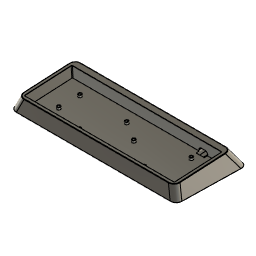
Menhirvan (Autodesk Fusion 360 design; units mm, degrees)
Autodesk Fusion 360 part; units mm, degrees
sketch "Top Plane Sketch" plane through (0, 0, 0) normal (0, 0, 1) x (1, 0, 0)
  line L0 (-95.25, -40.4812) -> (147.6375, -40.4812) construction
  line L1 (147.6375, -40.4812) -> (147.6375, 35.7188) construction
  line L2 (147.6375, 35.7188) -> (-95.25, 35.7188) construction
  line L3 (-95.25, 35.7188) -> (-95.25, -40.4813) construction
  line L4 (-95.75, -40.9812) -> (148.1375, -40.9812)
  line L5 (148.1375, -40.9812) -> (148.1375, 36.2188)
  line L6 (148.1375, 36.2188) -> (-95.75, 36.2188)
  line L7 (-95.75, 36.2188) -> (-95.75, -40.9812)
  line L8 (-100.75, -45.9812) -> (153.1375, -45.9812)
  line L9 (153.1375, -45.9812) -> (153.1375, 46.2188)
  line L10 (153.1375, 46.2188) -> (-100.75, 46.2188)
  line L11 (-100.75, 46.2188) -> (-100.75, -45.9812)
  line L12 (-95.25, 35.7188) -> (147.6375, -40.4813) construction
  line L13 (147.6375, 35.7188) -> (-95.25, -40.4813) construction
  circle A0 centre (26.1938, -2.3813) radius 1.8249 construction
  dimension "d1" = 242.8875
  dimension "d2" = 76.2
  dimension "d3" = 0.5
  dimension "d9" = 10
  dimension "d10" = 5
  dimension "d11" = 5
  dimension "d12" = 5
  constraint horizontal L0
  constraint vertical L1
  constraint horizontal L2
  constraint vertical L3
  constraint midpoint L12 A0.centre
  measures "d1" distance of L0.start L0.end
  measures "d2" distance of L0.start L2.end
  measures "d9" distance of L6 L10
  measures "d10" distance of L7 L11
  measures "d11" distance of L5 L9
  measures "d12" distance of L4 L8
ref_plane "WorkPlane1" through (0, 0, -50) normal (0, 0, 1) x (1, 0, 0)
sketch "Base Plane Sketch" plane through (0, 0, -50) normal (0, 0, 1) x (1, 0, 0)
  line L0 (147.6375, -35.7188) -> (-95.25, -35.7188) construction
  line L1 (-95.25, -35.7188) -> (-95.25, 40.4813) construction
  line L2 (-95.25, 40.4812) -> (147.6375, 40.4812) construction
  line L3 (147.6375, 40.4812) -> (147.6375, -35.7187) construction
  line L4 (147.6375, -35.7188) -> (-95.25, 40.4812) construction
  line L5 (-95.25, -35.7188) -> (147.6375, 40.4813) construction
  circle A0 centre (26.1938, 2.3812) radius 6.9017 construction
  line L6 (148.1375, -36.2188) -> (-95.75, -36.2188) construction
  line L7 (-95.75, -36.2188) -> (-95.75, 40.9812) construction
  line L8 (-95.75, 40.9812) -> (148.1375, 40.9812) construction
  line L9 (148.1375, 40.9812) -> (148.1375, -36.2188) construction
  line L10 (-100.75, 50.9812) -> (153.1375, 50.9812) construction
  line L11 (153.1375, 50.9812) -> (153.1375, -41.2188) construction
  line L12 (153.1375, -41.2188) -> (-100.75, -41.2188) construction
  line L13 (-100.75, -41.2188) -> (-100.75, 50.9812) construction
  line L14 (-120.75, 74.9813) -> (173.1375, 74.9813)
  line L15 (173.1375, 74.9813) -> (173.1375, -61.2188)
  line L16 (173.1375, -61.2188) -> (-120.75, -61.2188)
  line L17 (-120.75, -61.2188) -> (-120.75, 74.9813)
  point P0 (26.1938, 2.3812)
  dimension "d14" = 242.8875
  dimension "d15" = 76.2
  dimension "d16" = -0.5
  dimension "d17" = 10
  dimension "d18" = 5
  dimension "d19" = 5
  dimension "d20" = 5
  dimension "d21" = 20
  dimension "d22" = 20
  dimension "d23" = 20
  dimension "d24" = 24
  constraint horizontal L0
  constraint perpendicular L0 L1
  constraint parallel L0 L2
  constraint parallel L1 L3
  constraint coincident L4 P0
  constraint coincident L5 P0
  constraint coincident P0 A0.centre
  constraint horizontal L10
  constraint vertical L11
  constraint horizontal L12
  constraint vertical L13
  constraint horizontal L14
  constraint vertical L15
  constraint horizontal L16
  constraint vertical L17
  measures "d14" distance of L2.start L2.end
  measures "d15" distance of L0.end L2.start
  measures "d17" distance of L8 L10
  measures "d18" distance of L7 L13
  measures "d19" distance of L9 L11
  measures "d20" distance of L6 L12
  measures "d21" distance of L12 L16
  measures "d22" distance of L11 L15
  measures "d23" distance of L13 L17
  measures "d24" distance of L10 L14
loft "Loft1" add profiles "Top Plane Sketch", "Base Plane Sketch" section 1 section 2
sketch "Angle Cut Line" plane through (0, -42.0738, 12.822) normal (0, -0.956567, 0.291514) x (1, 0, 0)
  line L0 (153.1375, -13.4042) -> (-100.75, -13.4042)
  line L1 (-100.75, -13.4042) -> (-120.75, -65.6744)
  line L2 (-120.75, -65.6744) -> (173.1375, -65.6744)
  line L3 (173.1375, -65.6744) -> (153.1375, -13.4042)
  line L4 (-108.7852, -34.4042) -> (161.1727, -34.4042)
  dimension "d37" = 21
  constraint coincident L1 L4.start
  constraint coincident L3 L4.end
  constraint parallel L2 L4
  measures "d37" distance of L0 L4
ref_plane "WorkPlane2" through (26.1938, -52.103, -20.0879) normal (0, 0.052336, 0.99863) x (1, 0, 0)
extrude "Extrude1" cut 1 faces at (75.175, -15.8188, -50) along direction (0, 0, -1) up to surface end surface through (26.1938, -52.103, -20.0879) normal (0, 0.052336, 0.99863) offset 0
fillet "Fillet1" radius 10 4 edges at (-105.9551, 53.7043, -13.0127) (-104.7676, -49.0421, -10.0439) (157.1551, -49.0421, -10.0439) (158.3426, 53.7043, -13.0127)
extrude "Extrude2" cut sketch "Top Plane Sketch" against normal blind 18.06 contours L4 L5 L6 L7
sketch "USB C Hole" plane through (0, 36.2188, 0) normal (0, -1, 0) x (1, 0, 0)
  line L0 (-95.75, -18.06) -> (148.1375, -18.06)
  line L1 (124.347, -12.15) -> (110.397, -12.15)
  line L2 (110.397, -12.15) -> (110.397, -20.31)
  line L3 (110.397, -20.31) -> (124.347, -20.31)
  line L4 (124.347, -20.31) -> (124.347, -12.15)
  line L5 (124.347, -12.15) -> (110.397, -20.31) construction
  line L6 (110.397, -12.15) -> (124.347, -20.31) construction
  line L7 (148.1375, 0) -> (-95.75, 0)
  line L8 (-95.75, 0) -> (-95.75, -18.06)
  line L9 (148.1375, -18.06) -> (148.1375, 0)
  line L10 (-95.75, -18.06) -> (-86.225, -18.06) construction
  line L11 (-86.225, -18.06) -> (117.372, -18.06) construction
  line L12 (117.372, -18.06) -> (117.372, -16.23) construction
  point P0 (117.372, -16.23)
  dimension "d61" = 13.95
  dimension "d62" = 8.16
  dimension "d80" = 9.525
  dimension "d81" = 203.597
  dimension "d82" = 1.83
  constraint horizontal L1
  constraint perpendicular L1 L2
  constraint parallel L1 L3
  constraint parallel L2 L4
  constraint coincident L5 P0
  constraint coincident L6 P0
  constraint coincident L0.start L8.end
  constraint perpendicular L8 L10
  constraint parallel L0 L11
  constraint perpendicular L0 L12
  measures "d61" distance of L2.end L3.end
  measures "d62" distance of L1.end L2.end
  measures "d80" distance of L0.start L10.end
  measures "d81" distance of L10.end L11.end
  measures "d82" distance of L11.end P0
sketch "Screw Post Sketch" plane through (0, 0, -18.06) normal (0, 0, 1) x (1, 0, 0)
  circle A0 centre (-64.425, 17.1688) radius 2.75
  circle A1 centre (114.825, 19.2948) radius 2.75
  circle A2 centre (86.575, -29.3402) radius 2.75
  circle A3 centre (-66.025, -15.6052) radius 2.75
  circle A4 centre (-64.425, 17.1688) radius 1.6
  circle A5 centre (-66.025, -15.6052) radius 1.6
  circle A6 centre (114.825, 19.2948) radius 1.6
  circle A7 centre (86.575, -29.3402) radius 1.6
  line L0 (-95.75, -40.9812) -> (148.1375, -40.9812)
  line L1 (148.1375, -40.9812) -> (148.1375, 36.2188)
  line L2 (148.1375, 36.2188) -> (-95.75, 36.2188)
  line L3 (-95.75, 36.2188) -> (-95.75, -40.9812)
  line L4 (-95.75, 36.2188) -> (-86.225, 36.2188) construction
  line L5 (-86.225, 36.2188) -> (-86.225, 26.6938) construction
  line L6 (-86.225, 26.6938) -> (-95.75, 26.6938) construction
  line L7 (-95.75, 26.6938) -> (-95.75, 36.2188) construction
  circle A8 centre (-19.075, -29.0552) radius 2.75
  circle A9 centre (-19.075, -29.0552) radius 1.6
  circle A10 centre (42.425, -1.8812) radius 2.75
  circle A11 centre (42.425, -1.8812) radius 1.6
  circle A12 centre (11.775, 17.1688) radius 2.75
  circle A13 centre (11.775, 17.1688) radius 1.6
  dimension "d41" = 5.5
  dimension "d52" = 3.2
  dimension "d53" = 3.2
  dimension "d54" = 3.2
  dimension "d55" = 3.2
  dimension "d83" = 9.525
  dimension "d84" = 9.525
  dimension "d91" = 21.8
  dimension "d92" = 9.525
  dimension "d93" = 20.2
  dimension "d94" = 42.299
  dimension "d97" = 5.5
  dimension "d98" = 55.749
  dimension "d99" = 67.15
  dimension "d100" = 3.2
  dimension "d101" = 7.399
  dimension "d102" = 201.05
  dimension "d103" = 56.034
  dimension "d104" = 5.5
  dimension "d105" = 128.65
  dimension "d106" = 28.575
  dimension "d107" = 3.2
  dimension "d108" = 5.5
  dimension "d109" = 9.525
  dimension "d110" = 98
  dimension "d111" = 3.2
  dimension "d112" = 172.8
  constraint equal A0 A1
  constraint equal A0 A3
  constraint equal A0 A2
  constraint concentric A0 A4
  constraint concentric A3 A5
  constraint concentric A1 A6
  constraint concentric A2 A7
  constraint horizontal L4
  constraint vertical L5
  constraint horizontal L6
  constraint vertical L7
  constraint coincident L2.end L3.start
  constraint concentric A8 A9
  constraint concentric A10 A11
  constraint concentric A12 A13
  measures "d41" diameter of A0
  measures "d52" diameter of A4
  measures "d53" diameter of A5
  measures "d54" diameter of A6
  measures "d55" diameter of A7
  measures "d83" distance of L2.end L4.end
  measures "d84" distance of L2.end L6.end
  measures "d91" distance of A0.centre L5
  measures "d92" distance of A0.centre L6
  measures "d93" distance of A3.centre L5
  measures "d94" distance of A3.centre L6
  measures "d97" diameter of A8
  measures "d98" distance of L6 A8.centre
  measures "d99" distance of L5 A8.centre
  measures "d100" diameter of A9
  measures "d101" distance of A1.centre L6
  measures "d102" distance of A1.centre L5
  measures "d103" distance of A2.centre L6
  measures "d104" diameter of A10
  measures "d105" distance of L5 A10.centre
  measures "d106" distance of L6 A10.centre
  measures "d107" diameter of A11
  measures "d108" diameter of A12
  measures "d109" distance of L6 A12.centre
  measures "d110" distance of L5 A12.centre
  measures "d111" diameter of A13
  measures "d112" distance of A2.centre L5
fillet "Fillet2" radius 1 4 edges at (-95.75, 36.2188, -9.03) (148.1375, 36.2188, -9.03) (148.1375, -40.9812, -9.03) (-95.75, -40.9812, -9.03)
chamfer "Chamfer1" distance 0.5 angle 45 8 edges at (26.1938, -45.9812, 0) (150.3846, -43.3092, 0) (153.1375, 0.0798, 0) (150.6582, 43.5631, 0) (26.1937, 46.2188, 0) (-98.2707, 43.5631, 0) (-100.75, 0.0798, 0) (-97.9971, -43.3092, 0)
chamfer "Chamfer3" distance 0.25 angle 45 8 edges at (26.1938, 36.2188, 0) (147.8446, 35.9259, 0) (148.1375, -2.3812, 0) (147.8446, -40.6884, 0) (26.1938, -40.9812, 0) (-95.4571, -40.6884, 0) (-95.75, -2.3812, 0) (-95.4571, 35.9259, 0)
chamfer "Chamfer4" distance 0.5 angle 45 8 edges at (-109.9672, 4.2851, -23.0431) (-106.0874, -49.473, -20.2257) (26.1938, -52.103, -20.0879) (158.4749, -49.473, -20.2257) (162.3547, 4.2851, -23.0431) (161.0109, 58.4516, -25.8818) (26.1937, 61.1898, -26.0253) (-108.6234, 58.4516, -25.8818)
extrude "Extrude3" add sketch "Screw Post Sketch" along normal blind 3.46 contours A0 | A1 | A2 | A3 | A4 | A5 | A6 | A7 | A8 | A9 | A10 | A11 | A12 | A13
extrude "Extrude4" cut sketch "Screw Post Sketch" along normal blind 3.46 and the other way blind 0.54 contours A4 | A5 | A6 | A7 | A9 | A11 | A13
extrude "Extrude5" cut sketch "USB C Hole" along normal blind -25 and the other way blind -5 contours L0 L1 L2 L4 | L0 L2 L3 L4
fillet "Fillet3" radius 3.8 4 edges at (124.347, 44.5604, -20.31) (124.347, 44.7134, -12.15) (110.397, 44.5604, -20.31) (110.397, 44.7134, -12.15)
chamfer "Chamfer5" distance 0.25 angle 45 8 edges at (117.372, 53.208, -12.15) (111.51, 53.8483, -13.263) (110.397, 55.5551, -16.23) (111.51, 57.2618, -19.197) (117.372, 57.9021, -20.31) (123.234, 57.2618, -19.197) (124.347, 55.5551, -16.23) (123.234, 53.8483, -13.263)
move_body "Move2" bodies 1 to x (1, 0, 0) y (0, 0.99863, 0.052336) z (0, -0.052336, 0.99863) at (0, -1.1234, 2.6732)
equation "d1 = 19.05 mm * 12.75"
equation "d2 = 19.05 mm * 4"
equation "d14 = d1"
equation "d15 = d2"
equation "d17 = d9"
equation "d18 = d10"
equation "d19 = d11"
equation "d20 = d12"
equation "d21 = 10 mm * 2"
equation "d22 = d21"
equation "d23 = d21"
equation "d24 = 12 mm * 2"
equation "d25 = -3 deg"
equation "d53 = d52"
equation "d54 = d52"
equation "d55 = d52"
equation "d58 = 4 mm - 3.46 mm"
equation "d79 = -d25"
equation "d82 = ( 3.66 / 2 ) * 1 mm"
named bodies: "Bruce the Menhir"
